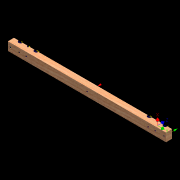
# Autodesk Inventor part: X_STRUCTURAL_SUP
Saved by Autodesk Inventor 2016 (Build 200138000, 138)
## iProperties
Created: 2016-07-06
Part Number: X_STRUCTURAL_SUP
Material: Wood (Birch)
Document SubType Name: Modeling
Designer: Jose
Density: 0.55 g/cm^3
Appearance: Birch - Natural Polished
Mass: 231.656 g
Surface Area: 708.586 cm^2
Volume: 421.192 cm^3
Author: Jose
Autodesk Inventor part; units mm, degrees
ref_plane "YZ Plane" through (0, 0, 0) normal (1, 0, 0) x (0, 1, 0)
ref_plane "XZ Plane" through (0, 0, 0) normal (0, 1, 0) x (-1, 0, 0)
ref_plane "XY Plane" through (0, 0, 0) normal (0, 0, 1) x (1, 0, 0)
sketch "Sketch1" plane through (0, 0, 0) normal (1, 0, 0) x (0, 1, 0)
  point P0 (0, 0)
sketch "Sketch2" plane through (0, 0, 0) normal (1, 0, 0) x (0, 1, 0)
  line L0 (11.5, 16) -> (-11.5, 16)
  line L1 (-11.5, 16) -> (-11.5, -16)
  line L2 (-11.5, -16) -> (11.5, -16)
  line L3 (11.5, -16) -> (11.5, 16)
  point P0 (0, 0)
  point P1 (11.5, 0)
  point P2 (0, 16)
  dimension "d0" = 32
  dimension "d1" = 23
  constraints: 8 end point, 2 midpoint, 2 parallel, 1 horizontal, 1 horizontal alignment, 1 perpendicular, 1 vertical alignment
  measures "d0" distance of L2.end L0.start
  measures "d1" distance of L1.end L2.end
extrude "Extrusion1" add sketch "Sketch2" along normal blind 600
sketch "Sketch3" plane through (0, -11.5, 16) normal (0, 0, 1) x (1, 0, 0)
  line L0 (0, 23) -> (0, 0) projected
  line L1 (0, 0) -> (600, 0) projected
  line L2 (600, 23) -> (600, 0) projected
  line L3 (0, 23) -> (600, 23) projected
  line L4 (0, 23) -> (600, 23) projected
  circle A0 centre (25, 23) radius 8.05
  circle A1 centre (85, 23) radius 8.05
  circle A2 centre (55, 23) radius 4.5
  line L5 (300, 23) -> (300, 0) construction
  circle A3 centre (575, 23) radius 8.05
  circle A4 centre (515, 23) radius 8.05
  circle A5 centre (545, 23) radius 4.5
  point P0 (0, 11.5)
  dimension "d4" = 60
  dimension "d5" = 30
  dimension "d6" = 16.1
  dimension "d7" = 25
  dimension "d8" = 9
  constraints: 6 centre point, 3 point on line, 3 symmetric about line, 2 end point, 2 midpoint, 1 equal radius, 3 other
  measures "d4" distance of A0.centre A1.centre
  measures "d5" distance of A1.centre A2.centre
  measures "d6" diameter of A1
  measures "d7" distance of L0.start A0.centre
  measures "d8" diameter of A2
extrude "Extrusion2" cut sketch "Sketch3" against normal through all contours A0 L3 | L3 A0 | A2 L3 | L3 A2 | A3 L3 | L3 A3 | A1 L3 | L3 A1 | A5 L3 | L3 A5 | A4 L3 | L3 A4
sketch "Sketch4" plane through (93.05, 11.5, -16) normal (0, 1, 0) x (1, 0, 0)
  line L0 (413.9, -32) -> (413.9, 0)
  line L1 (0, 0) -> (413.9, 0)
  line L2 (0, 0) -> (0, -32)
  line L3 (0, -32) -> (413.9, -32)
  line L4 (-16.1, -32) -> (-16.1, 0)
  line L5 (-33.55, 0) -> (-16.1, 0)
  line L6 (-33.55, 0) -> (-33.55, -32)
  line L7 (-33.55, -32) -> (-16.1, -32)
  line L8 (-42.55, -32) -> (-42.55, 0)
  line L9 (-60, 0) -> (-42.55, 0)
  line L10 (-60, 0) -> (-60, -32)
  line L11 (-60, -32) -> (-42.55, -32)
  line L12 (-76.1, -32) -> (-76.1, 0)
  line L13 (-93.05, 0) -> (-76.1, 0)
  line L14 (-93.05, 0) -> (-93.05, -32)
  line L15 (-93.05, -32) -> (-76.1, -32)
  line L16 (430, 0) -> (430, -32)
  line L17 (430, -32) -> (447.45, -32)
  line L18 (447.45, -32) -> (447.45, 0)
  line L19 (430, 0) -> (447.45, 0)
  line L20 (456.45, 0) -> (456.45, -32)
  line L21 (456.45, -32) -> (473.9, -32)
  line L22 (473.9, -32) -> (473.9, 0)
  line L23 (456.45, 0) -> (473.9, 0)
  line L24 (490, 0) -> (490, -32)
  line L25 (490, -32) -> (506.95, -32)
  line L26 (506.95, 0) -> (506.95, -32)
  line L27 (490, 0) -> (506.95, 0)
  line L28 (506.95, 0) -> (506.95, -32) construction
  line L29 (506.95, -16) -> (-93.05, -16) construction
  line L30 (-93.05, 0) -> (506.95, 0) construction
  line L31 (206.95, 0) -> (206.95, -32) construction
  circle A0 centre (498.475, -16) radius 3.25
  circle A1 centre (465.175, -16) radius 3.25
  circle A2 centre (438.725, -16) radius 3.25
  circle A3 centre (206.95, -16) radius 3.25
  circle A4 centre (-24.825, -16) radius 3.25
  circle A5 centre (-51.275, -16) radius 3.25
  circle A6 centre (-84.575, -16) radius 3.25
  point P0 (438.725, 0)
  point P1 (465.175, 0)
  point P2 (498.475, 0)
  point P3 (-84.575, 0)
  point P4 (-51.275, 0)
  point P5 (-24.825, 0)
extrude "Extrusion3" cut sketch "Sketch4" against normal through all contours A0 | A1 | A2 | A3 | A4 | A5 | A6
body "Solid1"
